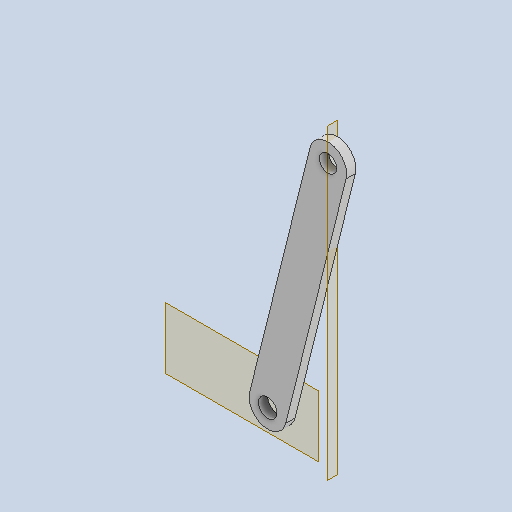
# Autodesk Inventor part: ramieR1
Saved by Autodesk Inventor 2025 (Build 290162000, 162)
## iProperties
Created: 2025-02-05
Part Number: ramieR1
Material: Generic
Document SubType Name: Modeling
Designer: piotr
Density: 1 g/cm^3
Appearance: Default
Author: piotr
Autodesk Inventor part; units mm, degrees
ref_plane "YZ Plane" through (0, 0, 0) normal (1, 0, 0) x (0, 1, 0)
ref_plane "XZ Plane" through (0, 0, 0) normal (0, 1, 0) x (-1, 0, 0)
ref_plane "XY Plane" through (0, 0, 0) normal (0, 0, 1) x (1, 0, 0)
ref_plane "Work Plane1" through (0, 0, 0) normal (0, 0, 1) x (1, 0, 0)
sketch "Sketch1" plane through (0, 0, 0) normal (0, 0, 1) x (1, 0, 0)
  circle A0 centre (112.5, -30) radius 10 projected
  circle A1 centre (112.5, -30) radius 20
  line L0 (112.5, -30) -> (177.3351, 230.0393)
  line L1 (112.5, -30) -> (380.5, -30) construction
  circle A2 centre (177.3351, 230.0393) radius 20
  line L2 (157.9292, 234.8777) -> (196.741, 225.2008)
  line L3 (93.0941, -25.1616) -> (131.9059, -34.8384)
  line L4 (93.0941, -25.1616) -> (131.9059, -34.8384)
  line L5 (131.9059, -34.8384) -> (196.741, 225.2008)
  line L6 (196.741, 225.2008) -> (157.9292, 234.8777)
  line L7 (157.9292, 234.8777) -> (93.0941, -25.1616)
  circle A3 centre (177.3351, 230.0393) radius 9.25
  point P0 (0, 0)
  dimension "d0" = 40
  dimension "d1" = 268
  dimension "d2" = 76
  dimension "d3" = 40
  dimension "d4" = 18.5
  dimension "d8" = 20
  constraints: 16 end point, 4 equal length, 4 point on circle, 3 centre point, 3 coincident, 3 perpendicular, 2 midpoint, 1 horizontal
  measures "d0" diameter of A1
  measures "d1" distance of L0.start L0.end
  measures "d2" angle of L1 L0
  measures "d3" diameter of A2
  measures "d4" diameter of A3
  measures "d8" diameter of A0
extrude "Extrusion1" add sketch "Sketch1" along normal blind 10 contours A0 L0 A1 L3 | A0 L3 A1 L0 | L3 A1 A0 | L0 A2 L5 A1 | A1 L7 A2 L0 | A2 L2 A3 L0 | L0 A3 L2 A2 | L2 A3 A2
ref_plane "Work Plane3" through (177.3351, 230.0393, 0) normal (1, 0, 0) x (0, 1, 0)
ref_plane "Work Plane2" through (150, -35, 30) normal (1, 0, 0) x (0, 1, 0)
body "Solid1"
